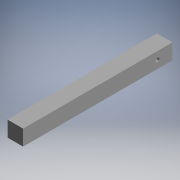
# Autodesk Inventor part: 30x30 pillars
Saved by Autodesk Inventor 2019 (Build 230136000, 136)
## iProperties
Part Number: 30x30 pillars
Material: Generic
Document SubType Name: Modeling
Designer: Delta
Appearance: Default
Author: Delta
Autodesk Inventor part; units mm, degrees
ref_plane "YZ Plane" through (0, 0, 0) normal (1, 0, 0) x (0, 1, 0)
ref_plane "XZ Plane" through (0, 0, 0) normal (0, 1, 0) x (-1, 0, 0)
ref_plane "XY Plane" through (0, 0, 0) normal (0, 0, 1) x (1, 0, 0)
sketch "Sketch1" plane through (0, 0, 0) normal (0, 0, 1) x (1, 0, 0)
  line L0 (0, 0) -> (31.75, 0)
  line L1 (31.75, 0) -> (31.75, 31.75)
  line L2 (31.75, 31.75) -> (0, 31.75)
  line L3 (0, 31.75) -> (0, 0)
  dimension "d0" = 31.75
  dimension "d1" = 31.75
  constraints: 8 end point, 2 parallel, 1 horizontal, 1 perpendicular
  measures "d0" distance between parallel lines of L1 L3
  measures "d1" distance between parallel lines of L0 L2
extrude "Extrusion1" add sketch "Sketch1" along normal blind 304.8
sketch "Sketch2" plane through (31.75, 0, 0) normal (1, 0, 0) x (0, 0, -1)
  line L0 (0, 0) -> (0, 31.75) projected
  line L1 (0, 31.75) -> (-304.8, 31.75) projected
  line L2 (0, 0) -> (-304.8, 0) projected
  circle A0 centre (-30.48, 15.875) radius 3.81
  dimension "d4" = 30.48
  dimension "d5" = 31.75
  dimension "d6" = 15.875
  dimension "d7" = 7.62
  constraints: 1 centre point, 1 coincident
  measures "d4" distance from line of L0 point (-30.48, 15.875)
  measures "d5" distance between parallel lines of L1 L2
  measures "d6" distance from line of L1 point (-30.48, 15.875)
  measures "d7" diameter of A0
extrude "Extrusion2" cut sketch "Sketch2" against normal through all
equation "\"d0\" = d1"
equation "\"d6\" = 0.5 * d5"
body "Solid1"
